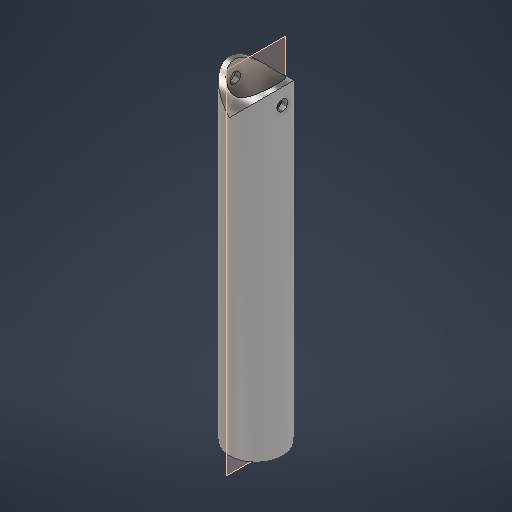
# Autodesk Inventor part: Steel rod
Saved by Autodesk Inventor 2026.2 (Build 302298010, 298A)
## iProperties
Created: 2026-04-01
Part Number: Steel rod
Material: Stainless Steel
Document SubType Name: Modeling
Designer: piete
Density: 8 g/cm^3
Appearance: Semi-Polished
Author: piete
Autodesk Inventor part; units mm, degrees
ref_plane "XZ Plane" through (0, 0, 0) normal (0, 1, 0) x (-1, 0, 0)
ref_plane "XY Plane" through (0, 0, 0) normal (0, 0, 1) x (1, 0, 0)
sketch "Sketch1" plane through (0, 0, 0) normal (0, 1, 0) x (-1, 0, 0)
  circle A0 centre (0, 0) radius 5
  circle A1 centre (0, 0) radius 4
  dimension "d0" = 10
  dimension "d1" = 8
  constraints: 2 centre point, 2 coincident
  measures "d0" diameter of A0
  measures "d1" diameter of A1
extrude "Extrusion1" add sketch "Sketch1" along normal blind 60
sketch "Sketch2" plane through (0, 0, 0) normal (1, 0, 0) x (0, 1, 0)
  circle A0 centre (57, 0) radius 1
  line L0 (60, -5) -> (60, 5) projected
  line L1 (0, -5) -> (0, 5) projected
  line L2 (0, -5) -> (60, -5) projected
  line L3 (60, -4) -> (0, -4) projected
  line L4 (60, 4) -> (0, 4) projected
  line L5 (0, 5) -> (60, 5) projected
  line L6 (60, 5) -> (57, 5)
  line L7 (60, 5) -> (60, -5)
  line L8 (57, -5) -> (60, -5)
  circle A1 centre (55, 0) radius 5
  point P0 (0, 0)
  point P1 (60, 0)
  point P2 (60, 0)
  point P3 (55, -5)
  point P4 (55, 5)
  dimension "d4" = 2
  dimension "d5" = 5
  dimension "d6" = 3
  dimension "d10" = 10
  dimension "d11" = 5
  dimension "d12" = 5
  constraints: 6 end point, 2 centre point, 2 point on line, 1 collinear, 1 midpoint, 1 perpendicular
  measures "d4" diameter of A0
  measures "d5" distance from line of L2 A0.centre
  measures "d6" distance from line of L0 A0.centre
  measures "d10" diameter of A1
  measures "d11" distance of point (60, 0) A1.centre
  measures "d12" distance from line of L6 A1.centre
extrude "Extrusion2" cut sketch "Sketch2" along normal through all both and the other way through all contours A0 | L2 A1 L3 L0 | L3 A1 L0 | A1 L4 L0 | L4 A1 L5 L0
body "Solid1"
